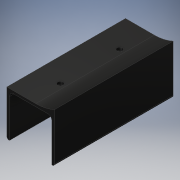
# Autodesk Inventor part: display_holder
Saved by Autodesk Inventor 2019.4 (Build 234330000, 330)
## iProperties
Created: 2020-09-30
Part Number: display_holder
Material: Generic
Document SubType Name: Modeling
Designer: deanv
Density: 1 g/cm^3
Appearance: Glossy - Black
Author: deanv
Autodesk Inventor part; units mm, degrees
ref_plane "YZ Plane" through (0, 0, 0) normal (1, 0, 0) x (0, 1, 0)
ref_plane "XZ Plane" through (0, 0, 0) normal (0, 1, 0) x (-1, 0, 0)
ref_plane "XY Plane" through (0, 0, 0) normal (0, 0, 1) x (1, 0, 0)
sketch "Sketch1" plane through (0, 0, 0) normal (0, 0, 1) x (1, 0, 0)
  line L0 (-20, -20) -> (20, -20)
  line L1 (20, -20) -> (20, 20)
  line L2 (20, 20) -> (-20, 20)
  line L3 (-20, 20) -> (-20, -20)
  line L4 (-20, -20) -> (20, 20) construction
  line L5 (20, -20) -> (-20, 20) construction
  line L6 (-22.5, 22.5) -> (22.5, 22.5)
  line L7 (22.5, 22.5) -> (22.5, -20)
  line L8 (22.5, -20) -> (-22.5, -20)
  line L9 (-22.5, -20) -> (-22.5, 22.5)
  line L10 (-33.9631, 22.5) -> (42.8206, 22.5) construction
  line L11 (-22.5, 22.5) -> (4.744, 22.5) construction
  line L12 (4.744, 22.5) -> (22.5, 22.5) construction
  line L13 (22.5, 22.5) -> (22.5, 26.484) construction
  line L14 (22.5, 26.484) -> (4.744, 26.484) construction
  line L15 (4.744, 26.484) -> (4.744, 22.5) construction
  arc A0 (4.744, 22.5) -> (22.5, 26.484) centre (4.7442, 64.059) ccw
  line L16 (22.5, 26.484) -> (22.5, 22.5)
  line L17 (22.5, 22.5) -> (4.744, 22.5)
  point P0 (0, 0)
  dimension "d0" = 40
  dimension "d1" = 40
  dimension "d2" = 2.5
  dimension "d3" = 42.5
  dimension "d4" = 2.5
  dimension "d5" = 2.5
  dimension "d6" = 27.244
  dimension "d7" = 3.984
  dimension "d8" = 41.559
  constraints: 36 end point, 6 parallel, 4 horizontal, 3 perpendicular, 2 collinear, 2 midpoint, 2 point on circle, 1 centre point, 1 point on line
  measures "d0" distance of L2.end L1.end
  measures "d1" distance of L1.end L0.end
  measures "d2" distance between parallel lines of L2 L6
  measures "d3" distance of L6.end L7.end
  measures "d4" distance between parallel lines of L1 L7
  measures "d5" distance between parallel lines of L3 L9
  measures "d6" distance of L6.start L11.end
  measures "d7" distance of L13.end L12.end
  measures "d8" radius of A0
extrude "Extrusion1" add sketch "Sketch1" along normal blind 112.1 contours L8 L9 L6 L7 L1 L2 L3 | L6 A0 L16
sketch "Sketch2" plane through (-20, 20, 0) normal (0, -1, 0) x (1, 0, 0)
  line L0 (0, 0) -> (0, 112.1) construction
  line L1 (40, 112.1) -> (40, 0) construction
  line L2 (0, 112.1) -> (40, 112.1) construction
  line L3 (40, 112.1) -> (40, 0) construction
  line L4 (40, 0) -> (0, 0) construction
  line L5 (0, 0) -> (0, 112.1) construction
  line L6 (20, 112.1) -> (20, 0) construction
  line L7 (24.744, 0) -> (24.744, 112.1) construction
  line L8 (42.5, 0) -> (40, 0) construction
  line L9 (0, 112.1) -> (40, 0) construction
  line L10 (0, 0) -> (40, 112.1) construction
  line L11 (40, 56.05) -> (0, 112.1) construction
  line L12 (0, 56.05) -> (40, 112.1) construction
  line L13 (0, 56.05) -> (40, 0) construction
  line L14 (40, 56.05) -> (0, 0) construction
  point P0 (20, 28.025)
  point P1 (20, 84.075)
  constraints: 22 end point, 5 midpoint, 5 parallel, 1 horizontal, 1 perpendicular
hole "Hole1" at (0, 20, 28.025) at (0, 20, 84.075) direction (0, 1, 0) diameter 5 depth 8 tip angle 118
fillet "Fillet1" radius 4 2 edges at (20, 20, 56.05) (-20, 20, 56.05)
fillet "Fillet2" radius 2 2 edges at (-22.5, -20, 56.05) (22.5, -20, 56.05)
equation "\"d4\" = d2"
equation "\"d5\" = d4"
body "Solid1"
